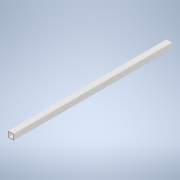
# Autodesk Inventor part: IgusDryLinQ-AWMQ-10
Saved by Autodesk Inventor 2020 (Build 240168000, 168)
## iProperties
Created: 2020-03-07
Part Number: IgusDryLinQ-AWMQ-10
Material: Aluminum 6061
Document SubType Name: Modeling
Designer: 10300812
Density: 2.7 g/cm^3
Appearance: Anodized - Light Gray
Author: 10300812
Autodesk Inventor part; units mm, degrees
ref_plane "YZ Plane" through (0, 0, 0) normal (1, 0, 0) x (0, 1, 0)
ref_plane "XZ Plane" through (0, 0, 0) normal (0, 1, 0) x (-1, 0, 0)
ref_plane "XY Plane" through (0, 0, 0) normal (0, 0, 1) x (1, 0, 0)
sketch "Sketch1" plane through (0, 0, 0) normal (0, 0, 1) x (1, 0, 0)
  circle A0 centre (0, 0) radius 5
  line L0 (-2.5, 2.5) -> (2.5, 2.5)
  line L1 (2.5, 2.5) -> (2.5, -2.5)
  line L2 (2.5, -2.5) -> (-2.5, -2.5)
  line L3 (-2.5, -2.5) -> (-2.5, 2.5)
  line L4 (-2.5, 2.5) -> (2.5, -2.5) construction
  line L5 (2.5, 2.5) -> (-2.5, -2.5) construction
  line L6 (-3.75, 3.75) -> (3.75, 3.75)
  line L7 (3.75, 3.75) -> (3.75, -3.75)
  line L8 (3.75, -3.75) -> (-3.75, -3.75)
  line L9 (-3.75, -3.75) -> (-3.75, 3.75)
  line L10 (-3.75, 3.75) -> (3.75, -3.75) construction
  line L11 (3.75, 3.75) -> (-3.75, -3.75) construction
  point P0 (-3.75, 3.3072)
  point P1 (-3.75, -3.3072)
  point P2 (-3.3072, -3.75)
  point P3 (3.3072, -3.75)
  point P4 (3.75, -3.3072)
  point P5 (3.75, 3.3072)
  point P6 (3.3072, 3.75)
  point P7 (-3.3072, 3.75)
  dimension "d0" = 10
  dimension "d1" = 5
  dimension "d2" = 5
  dimension "d3" = 7.5
  dimension "d4" = 7.5
  constraints: 24 end point, 4 midpoint, 4 parallel, 2 horizontal, 2 perpendicular, 1 centre point, 1 coincident
  measures "d0" diameter of A0
  measures "d1" distance of L1.end L2.end
  measures "d2" distance of L0.end L1.end
  measures "d3" distance of L7.end L8.end
  measures "d4" distance of L6.end L7.end
extrude "Extrusion1" add sketch "Sketch1" along normal blind 165 contours L7 A0 L8 L9 L6
body "Solid1"
